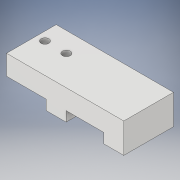
# Autodesk Inventor part: Load Cell holder
Saved by Autodesk Inventor 2019 (Build 230136000, 136)
## iProperties
Created: 2021-03-16
Part Number: Load Cell holder
Material: ABS Plastic
Document SubType Name: Modeling
Designer: User
Density: 1.06 g/cm^3
Appearance: Smooth - White
Author: User
Autodesk Inventor part; units mm, degrees
ref_plane "YZ Plane" through (0, 0, 0) normal (1, 0, 0) x (0, 1, 0)
ref_plane "XZ Plane" through (0, 0, 0) normal (0, 1, 0) x (-1, 0, 0)
ref_plane "XY Plane" through (0, 0, 0) normal (0, 0, 1) x (1, 0, 0)
sketch "Sketch1" plane through (0, 0, 0) normal (0, 0, 1) x (1, 0, 0)
  line L0 (0, 10) -> (0, 20)
  line L1 (0, 20) -> (59, 20)
  line L2 (59, 20) -> (59, 5)
  line L3 (59, 5) -> (49, 5)
  line L4 (49, 5) -> (49, 10)
  line L5 (49, 10) -> (30, 10)
  line L6 (30, 10) -> (30, 5)
  line L7 (30, 5) -> (20, 5)
  line L8 (20, 5) -> (20, 10)
  line L9 (20, 10) -> (0, 10)
  point P0 (0, 0)
  dimension "d0" = 19
  dimension "d1" = 10
  dimension "d2" = 10
  dimension "d3" = 20
  dimension "d4" = 10
  dimension "d5" = 5
  dimension "d6" = 59
  dimension "d7" = 10
  constraints: 20 end point, 5 perpendicular, 4 point on line, 1 vertical
  measures "d0" distance between parallel lines of L4 L6
  measures "d1" distance between parallel lines of L2 L4
  measures "d2" distance between parallel lines of L6 L8
  measures "d3" distance between parallel lines of L8 L0
  measures "d4" distance between parallel lines of L1 L9
  measures "d5" distance from line of L3.end L5
  measures "d6" distance from line of point (0, 0) L2
  measures "d7" distance from line of point (0, 0) L5
extrude "Extrusion1" add sketch "Sketch1" along normal mid plane 25
sketch "Sketch2" plane through (0, 20, 12.5) normal (0, 1, 0) x (1, 0, 0)
  circle A0 centre (4.3301, 15) radius 2
  circle A1 centre (15.1301, 15) radius 2
  line L0 (20, 25) -> (20, 0) projected
  line L1 (0, 25) -> (59, 25) projected
  point P0 (0, 12.5)
  dimension "d10" = 4
  dimension "d11" = 4
  dimension "d12" = 10.8
  dimension "d14" = 5
  dimension "d15" = 10
  dimension "d16" = 10
  constraints: 2 centre point
  measures "d10" diameter of A0
  measures "d11" diameter of A1
  measures "d12" distance of A0.centre A1.centre
  measures "d14" distance of A0.centre point (0, 12.5)
  measures "d15" distance from line of A0.centre L1
  measures "d16" distance from line of L1 A1.centre
extrude "Extrusion2" cut sketch "Sketch2" against normal blind 20
body "Solid1"
